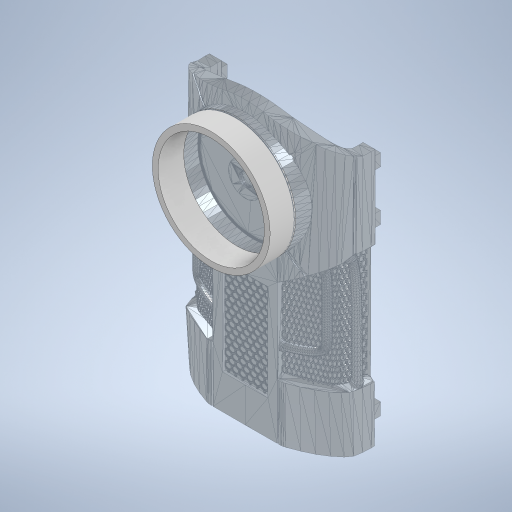
# Autodesk Inventor part: top_
Saved by Autodesk Inventor 2024.3 (Build 283343000, 343)
## iProperties
Created: 2025-07-23
Part Number: top_
Material: Genérico
Document SubType Name: Modeling
Designer: eliez
Density: 1 g/cm^3
Appearance: Valor por defecto
Author: eliez
Autodesk Inventor part; units mm, degrees
ref_plane "YZ Plane" through (0, 0, 0) normal (1, 0, 0) x (0, 1, 0)
ref_plane "XZ Plane" through (0, 0, 0) normal (0, 1, 0) x (-1, 0, 0)
ref_plane "Plano de trabajo1" through (3.0641, 65.4778, 24.5643) normal (0, 0, 1) x (1, 0, 0)
sketch "Boceto4" plane through (3.0641, 65.4778, 24.5643) normal (0, 0, 1) x (1, 0, 0)
  circle A0 centre (-2.8402, -28.9561) radius 32.1706 projected
  circle A1 centre (-2.8402, -28.9561) radius 29.0282
  point P0 (-3.0641, -65.4778)
  constraints: 1 centre point, 1 coincident
extrude "Extrusión2" add sketch "Boceto4" along normal blind 14
